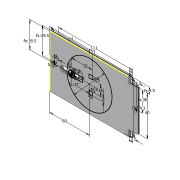
# Autodesk Inventor part: gps_cover_flat_only
Saved by Autodesk Inventor 2022 (Build 260153000, 153)
## iProperties
Created: 2022-05-19
Part Number: gps_cover_flat_only
Material: Generic
Document SubType Name: Modeling
Designer: Thomas
Density: 1 g/cm^3
Appearance: Default
Author: Thomas
Autodesk Inventor part; units mm, degrees
ref_plane "YZ Plane" through (0, 0, 0) normal (1, 0, 0) x (0, 1, 0)
ref_plane "XZ Plane" through (0, 0, 0) normal (0, 1, 0) x (-1, 0, 0)
ref_plane "XY Plane" through (0, 0, 0) normal (0, 0, 1) x (1, 0, 0)
sketch "Sketch1" plane through (0, 0, 0) normal (0, 0, 1) x (1, 0, 0)
  line L0 (0, 0) -> (123, 0)
  line L1 (123, 0) -> (123, 79)
  line L2 (123, 79) -> (0, 79)
  line L3 (0, 79) -> (0, 0)
  line L4 (12, 79) -> (12, 0)
  line L5 (123, 69.5) -> (126.5, 69.5)
  line L6 (126.5, 69.5) -> (126.5, 9.5)
  line L7 (126.5, 9.5) -> (123, 9.5)
  line L8 (123, 9.5) -> (123, 69.5)
  line L9 (126.5, 9.5) -> (132.5, 9.5)
  line L10 (132.5, 9.5) -> (132.5, 69.5)
  line L11 (132.5, 69.5) -> (126.5, 69.5)
  line L12 (126.5, 69.5) -> (126.5, 9.5)
  line L13 (123, 69.5) -> (119, 69.5)
  line L14 (119, 69.5) -> (119, 79)
  line L15 (119, 79) -> (123, 79)
  line L16 (123, 79) -> (123, 69.5)
  line L17 (123, 9.5) -> (119, 9.5)
  line L18 (119, 9.5) -> (119, 0)
  line L19 (119, 0) -> (123, 0)
  line L20 (123, 0) -> (123, 9.5)
  circle A0 centre (129.5, 39.5) radius 2.1
  line L21 (9, 39.5) -> (5, 39.5) construction
  line L22 (9, 42) -> (5, 42)
  line L23 (5, 37) -> (9, 37)
  arc A1 (9, 37) -> (9, 42) centre (9, 39.5) ccw
  arc A2 (5, 42) -> (5, 37) centre (5, 39.5) ccw
  point P0 (7, 39.5)
  dimension "d0" = 123
  dimension "d1" = 79
  dimension "d2" = 111
  dimension "d3" = 3.5
  dimension "d4" = 6
  dimension "d5" = 60
  dimension "d6" = 9.5
  dimension "d7" = 4
  dimension "d8" = 4
  dimension "d9" = 4.2
  dimension "d10" = 3
  dimension "d11" = 30
  dimension "d20" = 5
  dimension "d21" = 3
  dimension "d22" = 4
  dimension "d23" = 39.5
  constraints: 50 end point, 11 parallel, 6 horizontal, 6 perpendicular, 6 point on line, 4 point on circle, 4 tangent, 3 centre point, 1 midpoint
  measures "d0" distance of L2.end L1.end
  measures "d1" distance of L1.end L0.end
  measures "d2" distance between parallel lines of L4 L1
  measures "d3" distance of L6.end L7.end
  measures "d4" distance of L10.end L11.end
  measures "d5" distance of L9.end L10.end
  measures "d6" distance between parallel lines of L2 L11
  measures "d7" distance of L14.end L15.end
  measures "d8" distance of L19.end L18.end
  measures "d9" diameter of A0
  measures "d10" distance from line of L10 A0.centre
  measures "d11" distance from line of L11 A0.centre
  measures "d20" diameter of A2
  measures "d21" distance from line of L4 L21.start
  measures "d22" distance of L21.start L21.end
  measures "d23" distance from line of L2 point (7, 39.5)
extrude "Extrusion1" add sketch "Sketch1" along normal blind 2 contours L3 L2 L4 L0 | L4 L2 L14 L13 L1 L17 L18 L0 | L1 L5 L6 L7 | L6 L11 L10 L9 | A0
extrude "Extrusion3" add sketch "Sketch1" against normal blind 2 contours L4 L2 L14 L13 L1 L17 L18 L0 | L6 L11 L10 L9
sketch "Sketch2" plane through (0, 0, 2) normal (0, 0, 1) x (1, 0, 0)
  circle A0 centre (60, 39.5) radius 34
  line L0 (119, 79) -> (0, 79) projected
  line L1 (0, 79) -> (0, 0) projected
  line L2 (59, 52.5) -> (64, 52.5)
  line L3 (64, 52.5) -> (64, 47.5)
  line L4 (64, 47.5) -> (59, 47.5)
  line L5 (59, 47.5) -> (59, 52.5)
  line L6 (59, 31.5) -> (64, 31.5)
  line L7 (64, 31.5) -> (64, 26.5)
  line L8 (64, 26.5) -> (59, 26.5)
  line L9 (59, 26.5) -> (59, 31.5)
  circle A1 centre (33, 39.5) radius 1.5
  circle A2 centre (33, 39.5) radius 4
  line L10 (35, 42.9641) -> (35, 36.0359)
  line L11 (33, 41) -> (35, 41)
  line L12 (33, 38) -> (35, 38)
  circle A3 centre (33, 39.5) radius 5
  line L13 (35, 42.9641) -> (35, 44.0826)
  line L14 (35, 36.0359) -> (35, 34.9174)
  line L15 (35, 42.9641) -> (49, 42.9641)
  line L16 (49, 42.9641) -> (49, 36.0359)
  line L17 (49, 36.0359) -> (35, 36.0359)
  line L18 (35, 36.0359) -> (35, 42.9641)
  dimension "d24" = 68
  dimension "d25" = 39.5
  dimension "d26" = 60
  dimension "d27" = 16
  dimension "d28" = 5
  dimension "d29" = 5
  dimension "d30" = 8
  dimension "d31" = 5
  dimension "d32" = 31
  dimension "d33" = 27
  dimension "d34" = 3
  dimension "d35" = 8
  dimension "d36" = 64
  dimension "d37" = 2
  dimension "d38" = 10
  dimension "d51" = 16
  dimension "d52" = 6.9282
  constraints: 34 end point, 6 parallel, 6 point on circle, 5 perpendicular, 5 point on line, 4 centre point, 3 horizontal, 2 coincident, 2 tangent, 2 vertical
  measures "d24" diameter of A0
  measures "d25" distance from line of A0.centre L0
  measures "d26" distance from line of L1 A0.centre
  measures "d27" distance between parallel lines of L6 L4
  measures "d28" distance of L6.end L7.end
  measures "d29" distance of L2.end L3.end
  measures "d30" distance from line of A0.centre L6
  measures "d31" distance between parallel lines of L9 L7
  measures "d32" distance from line of L3 A1.centre
  measures "d33" distance of A1.centre A0.centre
  measures "d34" diameter of A1
  measures "d35" diameter of A2
  measures "d36" distance between parallel lines of L3 L1
  measures "d37" distance from line of A2.centre L10
  measures "d38" diameter of A3
  measures "d51" distance from line of A2.centre L16
  measures "d52" distance between parallel lines of L15 L17
extrude "Extrusion4" [suppressed]
sketch "Sketch3" plane through (0, 0, 5.7) normal (0, 0, 1) x (1, 0, 0)
  line L0 (59, 52.5) -> (64, 52.5) projected
  line L1 (59, 52.5) -> (65.1, 52.5)
  line L2 (65.1, 52.5) -> (65.1, 47.5)
  line L3 (65.1, 47.5) -> (59, 47.5)
  line L4 (59, 47.5) -> (59, 52.5)
  line L5 (59, 47.5) -> (64, 47.5) projected
  line L6 (59, 31.5) -> (64, 31.5) projected
  line L7 (59, 31.5) -> (65.1, 31.5)
  line L8 (65.1, 31.5) -> (65.1, 26.5)
  line L9 (65.1, 26.5) -> (59, 26.5)
  line L10 (59, 26.5) -> (59, 31.5)
  line L11 (59, 26.5) -> (64, 26.5) projected
  line L12 (64, 47.5) -> (64, 52.5) projected
  line L13 (64, 26.5) -> (64, 31.5) projected
  point P0 (0, 0)
  point P1 (61.5, 47.5)
  point P2 (61.5, 26.5)
  dimension "d41" = 1.1
  dimension "d42" = 1.1
  constraints: 16 end point, 4 parallel, 2 horizontal, 2 midpoint, 2 perpendicular, 2 point on line
  measures "d41" distance between parallel lines of L2 L12
  measures "d42" distance between parallel lines of L13 L8
extrude "Extrusion5" [suppressed]
fillet "Fillet1" [suppressed]
extrude "Extrusion6" [suppressed]
sketch "Sketch4" plane through (0, 0, 6.5) normal (0, 0, 1) x (1, 0, 0)
  line L0 (35, 42.9641) -> (35, 36.0359) projected
  line L1 (33, 41) -> (35, 41) projected
  circle A0 centre (33, 39.5) radius 1.5 projected
  line L2 (33, 38) -> (35, 38) projected
  arc A1 (35, 42.9641) -> (35, 36.0359) centre (33, 39.5) ccw projected
  point P0 (0, 0)
extrude "Extrusion7" [suppressed]
fillet "Fillet2" [suppressed]
extrude "Extrusion8" [suppressed]
fillet "Fillet3" [suppressed]
sketch "Sketch5" plane through (0, 0, 2) normal (0, 0, 1) x (1, 0, 0)
  point P0 (0, 0)
extrude "Extrusion9" cut sketch "Sketch1" along normal through all both and the other way through all contours A0
sketch "Sketch6" plane through (0, 0, 2) normal (0, 0, 1) x (1, 0, 0)
  line L0 (7, 39.5) -> (129.5, 39.5) construction
  line L1 (20, 39.5) -> (40, 39.5) construction
  line L2 (20, 35.5) -> (40, 35.5)
  line L3 (40, 43.5) -> (20, 43.5)
  arc A0 (20, 43.5) -> (20, 35.5) centre (20, 39.5) ccw
  arc A1 (40, 35.5) -> (40, 43.5) centre (40, 39.5) ccw
  line L4 (0, 79) -> (0, 0) projected
  point P0 (30, 39.5)
  dimension "d58" = 8
  dimension "d59" = 20
  dimension "d60" = 20
  constraints: 10 end point, 4 point on circle, 4 tangent, 2 centre point, 2 point on line, 1 horizontal, 1 midpoint, 1 parallel
  measures "d58" diameter of A1
  measures "d59" distance of L1.start L1.end
  measures "d60" distance from line of L4 L1.start
extrude "Extrusion10" cut sketch "Sketch6" against normal through all
equation "\"d6\" = -0.5 * d5 + 0.5 * d1"
equation "\"d10\" = 0.5 * d4"
equation "\"d11\" = 0.5 * d5"
equation "\"d23\" = 0.5 * d1"
equation "\"d25\" = d23"
equation "\"d29\" = d28"
equation "\"d30\" = 0.5 * d27"
body "Solid1"
